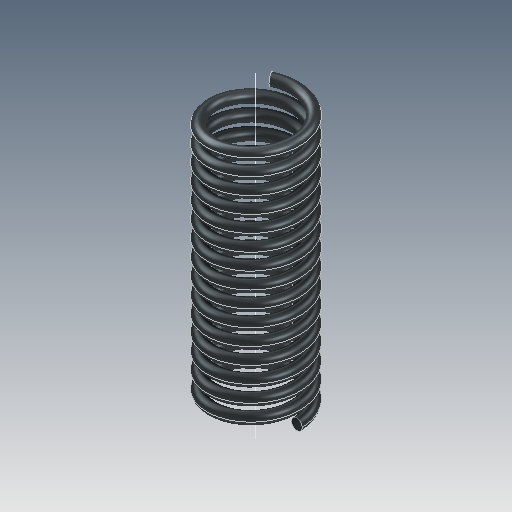
# Autodesk Inventor part: Resorte
Saved by Autodesk Inventor 2021 (Build 250183000, 183)
## iProperties
Created: 2024-03-17
Part Number: Resorte
Material: Iron, Ductile
Document SubType Name: Modeling
Designer: Martin
Density: 7.15 g/cm^3
Appearance: Iron Gray
Mass: 16.2306 g
Surface Area: 45.5092 cm^2
Volume: 2.27001 cm^3
Author: Martin
Autodesk Inventor part; units mm, degrees
ref_plane "YZ Plane" through (0, 0, 0) normal (1, 0, 0) x (0, 1, 0)
ref_plane "XZ Plane" through (0, 0, 0) normal (0, 1, 0) x (-1, 0, 0)
ref_plane "Work Plane1" through (0, 20, 0) normal (0, 1, 0) x (-1, 0, 0)
sketch "Sketch1" plane through (0, 0, 0) normal (0, 0, 1) x (1, 0, 0)
  circle A0 centre (7.5, 0) radius 1
  point P0 (0, 0)
  dimension "d0" = 2
  constraints: 1 centre point
  measures "d0" diameter of A0
coil "Coil1" sketch "Sketch1" operation add axis through (0, -10, 0) along (0, 1, 0) pitch 3 turns 15.333333 hand right
body "Solid1"
